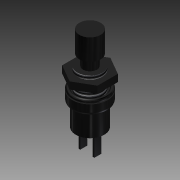
# Autodesk Inventor part: Pushbutton
Saved by Autodesk Inventor 2013 SP1 (Build 170176100, 176)
## iProperties
Created: 2012-12-09
Part Number: Pushbutton
Material: Allgemein
Document SubType Name: Modeling
Designer: Sebastian
Density: 1 g/cm^3
Author: Sebastian
Autodesk Inventor part; units mm, degrees
ref_plane "YZ Plane" through (0, 0, 0) normal (1, 0, 0) x (0, 1, 0)
ref_plane "XZ Plane" through (0, 0, 0) normal (0, 1, 0) x (-1, 0, 0)
ref_plane "XY Plane" through (0, 0, 0) normal (0, 0, 1) x (1, 0, 0)
sketch "Skizze1" plane through (0, 0, 0) normal (0, 0, 1) x (1, 0, 0)
  circle A0 centre (0, 0) radius 5
  dimension "d0" = 10
  constraints: 1 centre point, 1 coincident
  measures "d0" diameter of A0
extrude "Extrusion1" add sketch "Skizze1" against normal blind 3
fillet "Rundung1" radius 1 1 edges at (-5, 0, -3)
sketch "Skizze2" plane through (0, 0, 0) normal (0, 0, 1) x (1, 0, 0)
  circle A0 centre (0, 0) radius 3.5
  dimension "d4" = 7
  constraints: 1 centre point, 1 coincident
  measures "d4" diameter of A0
extrude "Extrusion2" add sketch "Skizze2" along normal blind 6
thread "Gewinde1" size "M7x1" class "6g" standard "ANSI Metric M Profile" full length
sketch "Skizze3" plane through (0, 0, 0) normal (0, 0, 1) x (1, 0, 0)
  circle A0 centre (0, 0) radius 2
  dimension "d9" = 4
  constraints: 1 centre point, 1 coincident
  measures "d9" diameter of A0
extrude "Extrusion3" add sketch "Skizze3" along normal blind 3 separate body
move or copy body "Körper verschieben1" bodies to move or copy 2 copy no translate (0, 0, 6)
sketch "Skizze4" plane through (0, 0, 0) normal (0, 0, 1) x (1, 0, 0)
  circle A0 centre (0, 0) radius 3
  dimension "d15" = 6
  constraints: 1 centre point, 1 coincident
  measures "d15" diameter of A0
extrude "Extrusion4" add sketch "Skizze4" along normal blind 6 separate body
move or copy body "Körper verschieben2" bodies to move or copy 3 copy no translate (0, 0, 9)
sketch "Skizze5" plane through (0, 0, 0) normal (0, 0, 1) x (1, 0, 0)
  circle A0 centre (0, 0) radius 4
  dimension "d21" = 8
  constraints: 1 centre point, 1 coincident
  measures "d21" diameter of A0
extrude "Extrusion5" add sketch "Skizze5" against normal blind 6 separate body
move or copy body "Körper verschieben3" bodies to move or copy 4 copy no translate (0, 0, -3)
sketch "Skizze6" plane through (0, 0, 0) normal (0, 0, 1) x (1, 0, 0)
  line L0 (-1.75, -1) -> (-2.25, -1)
  line L1 (-2.25, -1) -> (-2.25, 1)
  line L2 (-2.25, 1) -> (-1.75, 1)
  line L3 (-1.75, 1) -> (-1.75, -1)
  line L4 (-1.75, -1) -> (-2.25, 1) construction
  line L5 (-2.25, -1) -> (-1.75, 1) construction
  line L6 (1.75, -1) -> (2.25, -1)
  line L7 (2.25, -1) -> (2.25, 1)
  line L8 (2.25, 1) -> (1.75, 1)
  line L9 (1.75, 1) -> (1.75, -1)
  line L10 (1.75, -1) -> (2.25, 1) construction
  line L11 (2.25, -1) -> (1.75, 1) construction
  point P0 (0, 0)
  point P1 (-2, 0)
  point P2 (2, 0)
  dimension "d27" = 0.5
  dimension "d28" = 2
  dimension "d29" = 0.5
  dimension "d30" = 2
  constraints: 24 end point, 4 midpoint, 4 parallel, 2 horizontal, 2 perpendicular
  measures "d27" distance of L1.end L2.end
  measures "d28" distance of L0.end L1.end
  measures "d29" distance of L8.end L7.end
  measures "d30" distance of L7.end L6.end
extrude "Extrusion6" add sketch "Skizze6" against normal blind 6 separate body
move or copy body "Körper verschieben4" bodies to move or copy 5 copy no translate (0, 0, -9)
sketch "Skizze8" plane through (0, 0, 0) normal (0, 1, 0) x (-1, 0, 0)
  circle A0 centre (4.5, 0) radius 0.5
  line L0 (0, -1.125) -> (0, 1.125)
  line L1 (0, 0) -> (4.5, 0) construction
  dimension "d36" = 1
  dimension "d37" = 4.5
  constraints: 4 end point, 1 centre point, 1 horizontal, 1 perpendicular
  measures "d36" diameter of A0
  measures "d37" distance of L1.start L1.end
revolve "Umdrehung1" add sketch "Skizze8" angle 360 about axis through (0, 0, -1.125) along (0, 0, 1) separate body
move or copy body "Körper verschieben5" bodies to move or copy 6 copy no translate (0, 0, 0.5)
sketch "Skizze9" plane through (0, 0, 0) normal (0, 0, 1) x (1, 0, 0)
  line L0 (0, 5.7796) -> (5.0053, 2.8898)
  line L1 (5.0053, 2.8898) -> (5.0053, -2.8898)
  line L2 (5.0053, -2.8898) -> (0, -5.7796)
  line L3 (0, -5.7796) -> (-5.0053, -2.8898)
  line L4 (-5.0053, -2.8898) -> (-5.0053, 2.8898)
  line L5 (-5.0053, 2.8898) -> (0, 5.7796)
  circle A0 centre (0, 0) radius 3.5
  dimension "d44" = 7
  constraints: 12 end point, 2 coincident, 1 centre point, 13 other
  measures "d44" diameter of A0
extrude "Extrusion7" add sketch "Skizze9" along normal blind 2 separate body
move or copy body "Körper verschieben6" bodies to move or copy 7 copy no translate (0, 0, 3)
